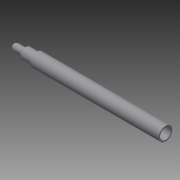
# Autodesk Inventor part: pen
Saved by Autodesk Inventor 2015 (Build 190159000, 159)
## iProperties
Created: 2014-11-30
Part Number: pen
Material: 常规
Document SubType Name: Modeling
Designer: zenkr
Density: 1 g/cm^3
Appearance: 默认
Author: zenkr
Autodesk Inventor part; units mm, degrees
ref_plane "YZ Plane" through (0, 0, 0) normal (1, 0, 0) x (0, 1, 0)
ref_plane "XZ Plane" through (0, 0, 0) normal (0, 1, 0) x (-1, 0, 0)
ref_plane "XY Plane" through (0, 0, 0) normal (0, 0, 1) x (1, 0, 0)
sketch "草图1" plane through (0, 0, 0) normal (1, 0, 0) x (0, 1, 0)
  circle A0 centre (0, 0) radius 5
  dimension "d0" = 10
  constraints: 1 centre point, 1 coincident
  measures "d0" diameter of A0
extrude "body" add sketch "草图1" along normal blind 94
sketch "草图2" plane through (0, 0, 0) normal (0, 0, 1) x (1, 0, 0)
  line L0 (0, 0) -> (0, 4)
  line L1 (0, 5) -> (0, -5) projected
  line L2 (0, 4) -> (-2, 4)
  line L3 (-2, 4) -> (-4, 4)
  line L4 (-4, 4) -> (-8, 4)
  line L5 (-8, 4) -> (-9.5, 2.5)
  line L6 (-9.5, 2.5) -> (-15.5, 2.5)
  line L7 (-15.5, 2.5) -> (-15.5, 2)
  line L8 (-15.5, 2) -> (-16.5, 2)
  line L9 (-16.5, 2) -> (-16.5, 0)
  line L10 (-18.0565, 0) -> (1.4122, 0)
  line L11 (-16.5, 0) -> (0, 0)
  dimension "d3" = 4
  dimension "d4" = 2
  dimension "d5" = 2
  dimension "d6" = 4
  dimension "d9" = 1.5
  dimension "d10" = 1.5
  dimension "d11" = 6
  dimension "d12" = 0.5
  dimension "d13" = 1
  constraints: 22 end point, 4 horizontal, 3 point on line, 2 perpendicular, 1 collinear, 1 vertical
  measures "d3" distance of L0.start L0.end
  measures "d4" distance of L0.end L2.end
  measures "d5" distance of L2.end L3.end
  measures "d6" distance of L3.end L4.end
  measures "d9" horizontal distance of L5.end L4.end
  measures "d10" horizontal distance of L4.end L5.end
  measures "d11" distance of L5.end L6.end
  measures "d12" distance of L6.end L7.end
  measures "d13" distance of L7.end L8.end
revolve "旋转1" add sketch "草图2" angle 360 about axis through (-18.0565, 0, 0) along (1, 0, 0)
shell "抽壳1" thickness 1 removed faces 2 at (94, -0.591, 1.5584) at (-16.5, 0.343, 0.4805)
